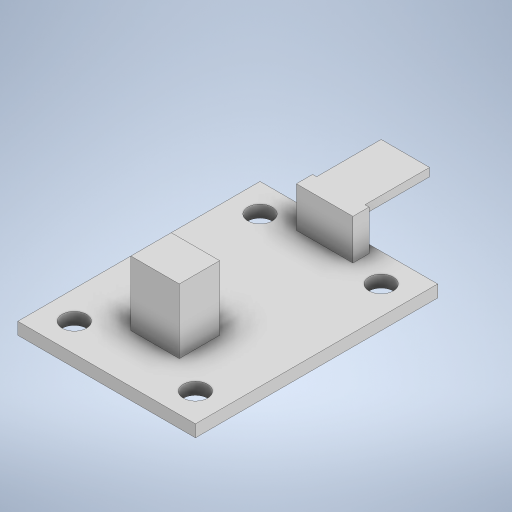
# Autodesk Inventor part: IR_Receiver
Saved by Autodesk Inventor 2024 (Build 280153000, 153)
## iProperties
Created: 2025-03-12
Part Number: IR_Receiver
Material: Generic
Document SubType Name: Modeling
Designer: 5454s
Density: 1 g/cm^3
Appearance: Default
Author: 5454s
Autodesk Inventor part; units mm, degrees
ref_plane "YZ Plane" through (0, 0, 0) normal (1, 0, 0) x (0, 1, 0)
ref_plane "XZ Plane" through (0, 0, 0) normal (0, 1, 0) x (-1, 0, 0)
ref_plane "XY Plane" through (0, 0, 0) normal (0, 0, 1) x (1, 0, 0)
sketch "Sketch1" plane through (0, 0, 0) normal (0, 1, 0) x (-1, 0, 0)
  line L0 (0, 0) -> (22, 0)
  line L1 (22, 0) -> (22, -30)
  line L2 (22, -30) -> (0, -30)
  line L3 (0, -30) -> (0, 0)
  circle A0 centre (18.5, -26.5) radius 1.5
  circle A1 centre (3.5, -26.5) radius 1.5
  circle A2 centre (3.5, -3.5) radius 1.5
  circle A3 centre (18.5, -3.5) radius 1.5
  line L4 (11, -30) -> (11, 0)
  line L5 (22, -15) -> (0, -15)
  dimension "d0" = 30
  dimension "d1" = 22
  dimension "d3" = 3
  dimension "d34" = 15
  dimension "d35" = 23
  dimension "d36" = 23
  dimension "d37" = 15
  constraints: 12 end point, 4 centre point, 4 midpoint, 3 equal radius, 2 parallel, 1 horizontal, 1 perpendicular, 2 other
  measures "d0" distance of L2.end L0.start
  measures "d1" distance of L0.start L0.end
  measures "d3" diameter of A0
  measures "d34" distance of A1.centre A0.centre
  measures "d35" distance of A3.centre A0.centre
  measures "d36" distance of A2.centre A1.centre
  measures "d37" distance of A2.centre A3.centre
extrude "Extrusion1" add sketch "Sketch1" along normal blind 1.5
sketch "Sketch2" plane through (0, 1.5, 0) normal (0, 1, 0) x (1, 0, 0)
  line L0 (-14.5, 27) -> (-7.5, 27)
  line L1 (-7.5, 27) -> (-7.5, 29)
  line L2 (-7.5, 29) -> (-14.5, 29)
  line L3 (-14.5, 29) -> (-14.5, 27)
  line L4 (0, 30) -> (-22, 30) projected
  line L5 (-22, 0) -> (0, 0) projected
  line L6 (-11, 0) -> (-11, 30)
  line L7 (-8, 6) -> (-14, 6)
  line L8 (-14, 6) -> (-14, 11)
  line L9 (-14, 11) -> (-8, 11)
  line L10 (-8, 11) -> (-8, 6)
  dimension "d14" = 7
  dimension "d15" = 2
  dimension "d16" = 1
  dimension "d20" = 5
  dimension "d21" = 6
  dimension "d22" = 6
  constraints: 18 end point, 4 parallel, 2 horizontal, 2 midpoint, 2 perpendicular, 2 other
  measures "d14" distance of L1.end L2.end
  measures "d15" distance of L0.end L1.end
  measures "d16" distance between parallel lines of L4 L2
  measures "d20" distance of L9.end L7.start
  measures "d21" distance of L7.start L7.end
  measures "d22" distance between parallel lines of L5 L7
extrude "Extrusion2" add sketch "Sketch2" along normal blind 8
sketch "Sketch3" plane through (-7.5, 1.5, -29) normal (0, 0, -1) x (-1, 0, 0)
  line L0 (0.5, 4) -> (6.5, 4)
  line L1 (6.5, 4) -> (6.5, 5)
  line L2 (6.5, 5) -> (0.5, 5)
  line L3 (0.5, 5) -> (0.5, 4)
  line L4 (-7.5, 0) -> (14.5, 0) projected
  line L5 (0, 0) -> (0, 8) projected
  line L6 (7, 0) -> (7, 8) projected
  point P0 (-7.5, -1.5)
  dimension "d25" = 4
  dimension "d26" = 6
  dimension "d27" = 1
  dimension "d28" = 0.5
  dimension "d29" = 0.5
  constraints: 8 end point, 2 parallel, 1 horizontal, 1 perpendicular
  measures "d25" distance between parallel lines of L4 L0
  measures "d26" distance of L0.start L0.end
  measures "d27" distance of L2.end L0.start
  measures "d28" distance between parallel lines of L5 L3
  measures "d29" distance between parallel lines of L6 L1
extrude "Extrusion3" add sketch "Sketch3" along normal blind 8
sketch "Sketch4" plane through (-7.5, 1.5, -29) normal (0, 0, -1) x (-1, 0, 0)
  line L0 (6.5, 5) -> (0.5, 5) projected
  line L1 (6.5, 4) -> (0.5, 4) projected
  line L2 (0.5, 4) -> (0.5, 5) projected
  line L3 (0.5, 5) -> (6.5, 5) projected
  line L4 (6.5, 5) -> (6.5, 4) projected
  line L5 (7, 0) -> (0, 0) projected
  line L6 (7, 0) -> (7, 8) projected
  line L7 (0, 8) -> (7, 8) projected
  line L8 (0, 0) -> (0, 8) projected
  line L9 (0, 5) -> (7, 5)
  point P0 (-7.5, -1.5)
  constraints: 3 point on line, 2 end point
extrude "Extrusion4" cut sketch "Sketch4" against normal blind 8 contours L0 L9 L8 L7 L6
body "Solid1"
